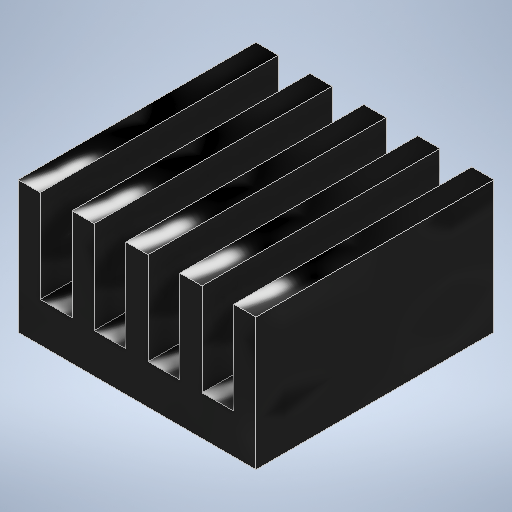
# Autodesk Inventor part: HEATSINK9x9
Saved by Autodesk Inventor 2025 (Build 290162000, 162)
## iProperties
Created: 2025-03-09
Part Number: HEATSINK9x9
Material: Aluminum 6061
Document SubType Name: Modeling
Designer: tvoko
Density: 2.7 g/cm^3
Appearance: Black
Author: tvoko
Autodesk Inventor part; units mm, degrees
ref_plane "YZ Plane" through (0, 0, 0) normal (1, 0, 0) x (0, 1, 0)
ref_plane "XZ Plane" through (0, 0, 0) normal (0, 1, 0) x (-1, 0, 0)
ref_plane "XY Plane" through (0, 0, 0) normal (0, 0, 1) x (1, 0, 0)
sketch "Sketch1" plane through (0, 0, 0) normal (0, 0, 1) x (1, 0, 0)
  line L0 (0, 0) -> (9, 0)
  line L1 (9, 0) -> (9, 5)
  line L2 (9, 5) -> (0, 5)
  line L3 (0, 5) -> (0, 0)
  line L4 (0.84, 5) -> (2.04, 5)
  line L5 (2.04, 5) -> (2.04, 1.5)
  line L6 (2.04, 1.5) -> (0.84, 1.5)
  line L7 (0.84, 1.5) -> (0.84, 5)
  line L8 (2.88, 5) -> (4.08, 5)
  line L9 (4.08, 5) -> (4.08, 1.5)
  line L10 (4.08, 1.5) -> (2.88, 1.5)
  line L11 (2.88, 1.5) -> (2.88, 5)
  line L12 (4.92, 5) -> (6.12, 5)
  line L13 (6.12, 5) -> (6.12, 1.5)
  line L14 (6.12, 1.5) -> (4.92, 1.5)
  line L15 (4.92, 1.5) -> (4.92, 5)
  line L16 (6.96, 5) -> (8.16, 5)
  line L17 (8.16, 5) -> (8.16, 1.5)
  line L18 (8.16, 1.5) -> (6.96, 1.5)
  line L19 (6.96, 1.5) -> (6.96, 5)
  line L20 (8.16, 3.25) -> (9, 3.25) construction
  line L21 (6.96, 3.25) -> (6.12, 3.25) construction
  line L22 (4.92, 3.25) -> (4.08, 3.25) construction
  line L23 (2.88, 3.25) -> (2.04, 3.25) construction
  line L24 (0.84, 3.25) -> (0, 3.25) construction
  dimension "d0" = 9
  dimension "d2" = 5
  dimension "d3" = 1.2
  dimension "d4" = 3.5
  constraints: 50 end point, 10 parallel, 9 point on line, 8 midpoint, 7 collinear, 7 perpendicular, 5 horizontal
  measures "d0" distance of L1.end L2.end
  measures "d2" distance of L0.end L1.end
  measures "d3" distance of L5.end L6.end
  measures "d4" distance of L6.end L4.start
extrude "Extrusion1" add sketch "Sketch1" along normal blind 9 contours L3 L2 L7 L6 L5 L11 L10 L9 L15 L14 L13 L19 L18 L17 L1 L0
body "Solid1"
